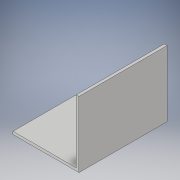
# Autodesk Inventor part: lifterMount
Saved by Autodesk Inventor 2017 (Build 210142000, 142)
## iProperties
Created: 2017-02-01
Part Number: lifterMount
Material: Generic
Document SubType Name: Modeling
Designer: kingb
Density: 1 g/cm^3
Appearance: Default
Author: kingb
Autodesk Inventor part; units mm, degrees
ref_plane "YZ Plane" through (0, 0, 0) normal (1, 0, 0) x (0, 1, 0)
ref_plane "XZ Plane" through (0, 0, 0) normal (0, 1, 0) x (-1, 0, 0)
ref_plane "XY Plane" through (0, 0, 0) normal (0, 0, 1) x (1, 0, 0)
sketch "Sketch1" plane through (0, 0, 0) normal (0, 0, 1) x (1, 0, 0)
  line L0 (0, 0) -> (-152.4, 0)
  line L1 (0, 0) -> (0, 152.4)
  line L2 (0, 152.4) -> (-6.35, 152.4)
  line L3 (-152.4, 0) -> (-152.4, 6.35)
  line L4 (-152.4, 6.35) -> (-6.35, 6.35)
  line L5 (-6.35, 6.35) -> (-6.35, 152.4)
  dimension "d0" = 152.4
  dimension "d1" = 152.4
  dimension "d2" = 6.35
  dimension "d3" = 6.35
  constraints: 12 end point, 3 perpendicular, 1 horizontal, 1 parallel, 1 vertical
  measures "d0" distance of L0.start L0.end
  measures "d1" distance of L0.start L1.end
  measures "d2" distance of L1.end L2.end
  measures "d3" distance of L0.end L3.end
extrude "Extrusion1" add sketch "Sketch1" along normal blind 203.2
body "Solid1"
